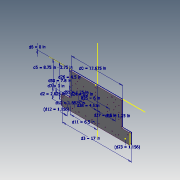
# Autodesk Inventor part: J005209
Saved by Autodesk Inventor 2015 SP1 (Build 190203100, 203)
## iProperties
Created: 2015-05-13
Material: Generic
Vendor: HHMI: JRC - ID&F
Document SubType Name: Modeling
Designer: ARNOLDJ
Density: 1 g/cm^3
Appearance: Default
Part Number: J005209
Description: REGULATOR BASE PLATE
RuleStatus: InUse
AfterDocSave0: file://Part Number Cleaner
DESIGN DEPARTMENT: HHMI: JRC - ID&F
ALTERED ITEM PART NUMBER: N/A
ALTERED ITEM VENDOR: N/A
ALTERED ITEM DESCRIPTION: N/A
Revision Number: 0
Autodesk Inventor part; units mm, degrees
ref_plane "YZ Plane" through (0, 0, 0) normal (1, 0, 0) x (0, 1, 0)
ref_plane "XZ Plane" through (0, 0, 0) normal (0, 1, 0) x (-1, 0, 0)
ref_plane "XY Plane" through (0, 0, 0) normal (0, 0, 1) x (1, 0, 0)
sketch "Sketch1" plane through (0, 0, 0) normal (0, 0, 1) x (1, 0, 0)
  line L0 (160.3375, -152.4) -> (-160.3375, -152.4)
  line L1 (-160.3375, -152.4) -> (-160.3375, 0)
  line L2 (-160.3375, 0) -> (160.3375, 0)
  line L3 (160.3375, 0) -> (160.3375, -152.4)
  line L4 (0, 223.4715) -> (0, -292.8328) projected
  line L5 (-302.26, 0) -> (302.26, 0) projected
  line L6 (215.9, -219.075) -> (-215.9, -219.075)
  line L7 (-215.9, -219.075) -> (-215.9, -152.4)
  line L8 (-215.9, -152.4) -> (215.9, -152.4)
  line L9 (215.9, -152.4) -> (215.9, -219.075)
  line L10 (215.9, -219.075) -> (-215.9, -152.4) construction
  line L11 (-215.9, -219.075) -> (215.9, -152.4) construction
  line L12 (0, 0) -> (0, 149.7138) construction
  line L13 (-143.6687, -198.12) -> (-186.5312, -198.12) construction
  line L14 (76.2, -105.41) -> (-76.2, -105.41) construction
  line L15 (-76.2, -105.41) -> (-76.2, -123.19) construction
  line L16 (-76.2, -123.19) -> (76.2, -123.19) construction
  line L17 (76.2, -123.19) -> (76.2, -105.41) construction
  line L18 (76.2, -105.41) -> (-76.2, -123.19) construction
  line L19 (-76.2, -105.41) -> (76.2, -123.19) construction
  point P0 (0, -185.7375)
  point P1 (-165.1, -198.12)
  point P2 (0, -114.3)
  point P3 (114.3, -114.3)
  point P4 (-114.3, -114.3)
  point P5 (0, -114.3)
  point P6 (-146.05, -114.3)
  point P7 (146.05, -114.3)
  point P8 (0, -114.3)
  point P9 (0, -114.3)
  dimension "d0" = 320.675
  dimension "d2" = 66.675
  dimension "d3" = 431.8
  dimension "d5" = 152.4
  dimension "d6" = 0
  dimension "d7" = 0
  dimension "d10" = 42.8625
  dimension "d11" = 165.1
  dimension "d12" = 29.3687
  dimension "d24" = 17.78
  dimension "d25" = 152.4
  dimension "d26" = 114.3
  dimension "d27" = 114.3
  dimension "d28" = 114.3
  dimension "d50" = 198.12
  dimension "d55" = 31.75
  dimension "d56" = 31.75
  constraints: 36 end point, 7 midpoint, 6 parallel, 5 horizontal alignment, 4 horizontal, 3 coincident, 3 perpendicular, 3 point on line, 1 other
  measures "d0" distance of L0.start L0.end
  measures "d2" distance of L6.end L7.end
  measures "d3" distance of L6.start L6.end
  measures "d5" distance of L0.end L1.end
  measures "d6" distance between parallel lines of L2 L5
  measures "d7" distance between parallel lines of L8 L0
  measures "d10" distance of L13.end L13.start
  measures "d11" distance from line of point (-165.1, -198.12) L12
  measures "d12" distance from line of L7 L13.end
  measures "d24" distance of L14.end L15.end
  measures "d25" distance of L14.start L14.end
  measures "d26" distance from line of L5 point (0, -114.3)
  measures "d27" distance of point (0, -114.3) point (114.3, -114.3)
  measures "d28" distance of point (0, -114.3) point (-114.3, -114.3)
  measures "d50" distance from line of L5 L13.end
  measures "d55" distance of point (-114.3, -114.3) point (-146.05, -114.3)
  measures "d56" distance of point (146.05, -114.3) point (114.3, -114.3)
extrude "Extrusion1" add sketch "Sketch1" along normal blind 9.144
hole "Hole1-Regulator Brkt Mtg" at (-186.5312, -198.12, 0) at (-143.6687, -198.12, 0) direction (0, 0, 1) diameter 4.1402 end through all
pattern_linear "Rectangular Pattern1" count 5 spacing 82.55 along (1, 0, 0) of "Hole1-Regulator Brkt Mtg"
sketch "Sketch2" plane through (0, 0, 9.144) normal (0, 0, 1) x (1, 0, 0)
  circle A0 centre (186.5313, -198.12) radius 2.0701 projected
  line L0 (215.9, -219.075) -> (215.9, -152.4) projected
  point P0 (0, 0)
  dimension "d23" = 29.3687
  measures "d23" distance from line of L0 A0.centre
hole "Hole2-Manifold Mtg" at (-114.3, -114.3, 0) at (-76.2, -123.19, 0) at (76.2, -105.41, 0) at (114.3, -114.3, 0) at (0, -114.3, 0) at (-146.05, -114.3, 0) at (146.05, -114.3, 0) direction (0, 0, 1) diameter 3.2512 end through all
sketch "Sketch3" plane through (0, 0, 0) normal (0, 0, 1) x (1, 0, 0)
  line L0 (-101.6, -15.24) -> (101.6, -15.24) construction
  line L1 (-203.2, -167.64) -> (203.2, -167.64) construction
  line L2 (0, 0) -> (0, 149.7138) construction
  line L3 (0, 223.4715) -> (0, -292.8328) construction
  line L4 (-287.02, 0) -> (299.72, 0) construction
  point P0 (0, -15.24)
  point P1 (0, -167.64)
  dimension "d36" = 101.6
  dimension "d37" = 101.6
  dimension "d38" = 15.24
  dimension "d39" = 203.2
  dimension "d40" = 406.4
  dimension "d41" = 152.4
  dimension "d54" = 152.4
  constraints: 4 end point, 2 horizontal, 2 point on line, 1 midpoint
  measures "d36" distance from line of L3 L0.start
  measures "d37" distance from line of L3 L0.end
  measures "d38" distance from line of L4 L0.start
  measures "d39" distance from line of L2 L1.start
  measures "d40" distance of L1.end L1.start
  measures "d41" vertical distance of L1.start L0.start
  measures "d54" distance of point (0, -15.24) point (0, -167.64)
hole "Hole3-Mount to Base plate" at (-101.6, -15.24, 0) at (101.6, -15.24, 0) at (203.2, -167.64, 0) at (-203.2, -167.64, 0) at (0, -15.24, 0) at (0, -167.64, 0) direction (0, 0, 1) diameter 7.493 end through all
fillet "Fillet1" radius 6.35 8 edges at (-215.9, -219.075, 4.572) (215.9, -219.075, 4.572) (160.3375, 0, 4.572) (160.3375, -152.4, 4.572) (215.9, -152.4, 4.572) (-215.9, -152.4, 4.572) (-160.3375, -152.4, 4.572) (-160.3375, 0, 4.572)
pattern_linear "Rectangular Pattern2" count 3 spacing 38.1 along (0, 1, 0) of "Hole2-Manifold Mtg"
sketch "Sketch4" plane through (0, 0, 0) normal (0, 0, 1) x (1, 0, 0)
  circle A0 centre (-143.6687, -198.12) radius 2.0701 projected
  circle A1 centre (-103.9812, -198.12) radius 2.0701 projected
  circle A2 centre (-143.6687, -198.12) radius 2.0701 construction
  circle A3 centre (-103.9812, -198.12) radius 2.0701 construction
  line L0 (-143.6687, -198.12) -> (-103.9812, -198.12) construction
  line L1 (-123.8599, -207.645) -> (-123.825, -198.12) construction
  line L2 (0, 43.815) -> (0, -262.89) projected
  point P0 (0, 0)
  point P1 (-123.8599, -55.245)
  point P2 (-123.8599, -17.145)
  dimension "d57" = 152.4
  dimension "d58" = 38.1
  dimension "d66" = 9.525
  dimension "d67" = 123.8599
  constraints: 4 end point, 1 horizontal, 1 midpoint
  measures "d57" distance of point (-123.86, -55.245) L1.start
  measures "d58" distance of point (-123.86, -55.245) point (-123.86, -17.145)
  measures "d66" distance from line of L0 L1.start
  measures "d67" distance from line of L2 L1.start
hole "Hole4-trough mounting" at (-123.8599, -17.145, 0) at (-123.8599, -55.245, 0) at (-123.8599, -207.645, 0) direction (0, 0, 1) diameter 3.2512 end through all
mirror "Mirror1" about plane through (0, 0, 0) normal (1, 0, 0) of "Hole4-trough mounting"
pattern_linear "Rectangular Pattern3" count 2 spacing 123.8504 along (1, 0, 0) of "Hole4-trough mounting"
body "Solid1"
